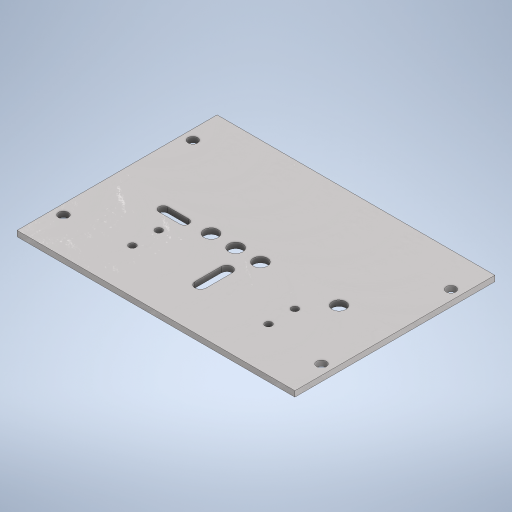
# Autodesk Inventor part: dach
Saved by Autodesk Inventor 2023 (Build 270158000, 158)
## iProperties
Created: 2023-07-07
Part Number: dach
Material: Stal miękka, spawana
Document SubType Name: Modeling
Designer: Kamil
Density: 7.85 g/cm^3
Appearance: Spawane — stal miękka
Author: Kamil
Autodesk Inventor part; units mm, degrees
ref_plane "YZ Plane" through (0, 0, 0) normal (1, 0, 0) x (0, 1, 0)
ref_plane "XZ Plane" through (0, 0, 0) normal (0, 1, 0) x (-1, 0, 0)
ref_plane "XY Plane" through (0, 0, 0) normal (0, 0, 1) x (1, 0, 0)
sketch "Szkic1" plane through (0, 0, 0) normal (0, 1, 0) x (-1, 0, 0)
  line L0 (0, 0) -> (-100, 0)
  line L1 (-100, 0) -> (-100, -70)
  line L2 (-100, -70) -> (0, -70)
  line L3 (0, -70) -> (0, 0)
  dimension "d0" = 100
  dimension "d1" = 70
  constraints: 8 end point, 2 parallel, 1 horizontal, 1 perpendicular
  measures "d0" distance of L2.end L1.end
  measures "d1" distance of L1.end L0.end
extrude "Wyciągnięcie proste1" add sketch "Szkic1" along normal blind 0.5
sketch "Szkic2" plane through (0, 0.5, 0) normal (0, 1, 0) x (1, 0, 0)
  line L0 (84.2801, 35.4995) -> (78.4801, 35.4995) projected
  line L1 (84.3801, 29.5995) -> (84.3801, 35.3995) projected
  line L2 (78.4801, 29.4995) -> (84.2801, 29.4995) projected
  line L3 (78.3801, 35.3995) -> (78.3801, 29.5995) projected
  circle A0 centre (53.6914, 31.8917) radius 2.05 projected
  circle A1 centre (44.8014, 31.8917) radius 2.05 projected
  circle A2 centre (35.9114, 31.8917) radius 2.05 projected
  line L4 (27.6783, 30.5334) -> (27.6783, 31.1734) projected
  line L5 (19.4183, 31.1734) -> (19.4183, 30.5334) projected
  line L6 (84.3801, 29.4995) -> (78.3801, 29.4995)
  line L7 (78.3801, 29.4995) -> (78.3801, 35.4995)
  line L8 (78.3801, 35.4995) -> (84.3801, 35.4995)
  line L9 (84.3801, 35.4995) -> (84.3801, 29.4995)
  line L10 (84.8801, 28.9995) -> (77.8801, 28.9995)
  line L11 (77.8801, 28.9995) -> (77.8801, 35.9995)
  line L12 (77.8801, 35.9995) -> (84.8801, 35.9995)
  line L13 (84.8801, 35.9995) -> (84.8801, 28.9995)
  circle A3 centre (53.6914, 31.8917) radius 2.55
  circle A4 centre (44.8014, 31.8917) radius 2.55
  circle A5 centre (35.9114, 31.8917) radius 2.55
  line L14 (27.6783, 30.5334) -> (19.4183, 30.5334)
  line L15 (19.4183, 30.5334) -> (19.4183, 31.1734)
  line L16 (19.4183, 31.1734) -> (27.6783, 31.1734)
  line L17 (27.6783, 31.1734) -> (27.6783, 30.5334)
  line L18 (28.9783, 32.4734) -> (18.1183, 32.4734)
  line L19 (18.1183, 32.4734) -> (18.1183, 29.2334)
  line L20 (18.1183, 29.2334) -> (28.9783, 29.2334)
  line L21 (28.9783, 29.2334) -> (28.9783, 32.4734)
  point P0 (0, 0)
  dimension "d4" = 0.5
  dimension "d5" = 0.5
  dimension "d6" = 0.5
  dimension "d7" = 0.5
  dimension "d8" = 1.3
  constraints: 32 end point, 8 parallel, 4 perpendicular, 3 centre point, 2 horizontal, 6 other
  measures "d4" distance between parallel lines of L9 L13
  measures "d5" radial gap between concentric circles of A0 A3
  measures "d6" radial gap between concentric circles of A1 A4
  measures "d7" radial gap between concentric circles of A2 A5
  measures "d8" distance between parallel lines of L16 L18
extrude "Wyciągnięcie proste2" cut sketch "Szkic2" against normal through all contours L8 L9 L1 L6 L2 L7 L3 L0 | A0 | A1 | A2 | L14 L5 L16 L4 | L10 L11 L12 L13 | A3 | A4 | A5 | L21 L20 L19 L18
sketch "Szkic3" plane through (0, 0.5, 0) normal (0, 1, 0) x (1, 0, 0)
  circle A0 centre (3.55, 57.7319) radius 1.5 projected
  circle A1 centre (3.55, 11.1233) radius 1.5 projected
  circle A2 centre (96.45, 57.7319) radius 1.5 projected
  circle A3 centre (96.45, 11.1233) radius 1.5 projected
  circle A4 centre (25.5, 23.5) radius 1 projected
  circle A5 centre (25.5, 14) radius 1 projected
  circle A6 centre (50, 23.5) radius 1 projected
  circle A7 centre (50, 14) radius 1 projected
  circle A8 centre (74.5, 23.5) radius 1 projected
  circle A9 centre (74.5, 14) radius 1 projected
  point P0 (0, 0)
extrude "Wyciągnięcie proste3" cut sketch "Szkic3" against normal through all
sketch "Szkic4" plane through (0, 0.5, 0) normal (0, 1, 0) x (1, 0, 0)
  circle A0 centre (3.55, 57.7319) radius 1.5 projected
  circle A1 centre (50, 14) radius 1 projected
  circle A2 centre (74.5, 14) radius 1 projected
  circle A3 centre (25.5, 23.5) radius 1 projected
  circle A4 centre (96.45, 57.7319) radius 1.5 projected
  circle A5 centre (3.55, 11.1233) radius 1.5 projected
  circle A6 centre (50, 23.5) radius 1 projected
  circle A7 centre (74.5, 23.5) radius 1 projected
  circle A8 centre (25.5, 14) radius 1 projected
  circle A9 centre (96.45, 11.1233) radius 1.5 projected
  circle A10 centre (44.8014, 31.8917) radius 2.55 projected
  circle A11 centre (35.9114, 31.8917) radius 2.55 projected
  circle A12 centre (53.6914, 31.8917) radius 2.55 projected
  line L0 (28.9783, 29.2334) -> (18.1183, 29.2334) projected
  line L1 (18.1183, 29.2334) -> (18.1183, 32.4734) projected
  line L2 (18.1183, 32.4734) -> (28.9783, 32.4734) projected
  line L3 (28.9783, 32.4734) -> (28.9783, 29.2334) projected
  line L4 (77.8801, 28.9995) -> (77.8801, 35.9995) projected
  line L5 (77.8801, 35.9995) -> (84.8801, 35.9995) projected
  line L6 (84.8801, 35.9995) -> (84.8801, 28.9995) projected
  line L7 (84.8801, 28.9995) -> (77.8801, 28.9995) projected
  line L8 (100, 0) -> (100, 70) projected
  line L9 (100, 70) -> (0, 70) projected
  line L10 (0, 70) -> (0, 0) projected
  line L11 (0, 0) -> (100, 0) projected
extrude "Wyciągnięcie proste4" add sketch "Szkic4" along normal blind 1.2
sketch "Szkic5" plane through (0, 1.7, 0) normal (0, 1, 0) x (1, 0, 0)
  circle A0 centre (25.5, 14) radius 1 projected
  line L0 (100, 70) -> (0, 70) projected
  line L1 (0, 70) -> (0, 0) projected
  line L2 (0, 0) -> (100, 0) projected
  line L3 (100, 0) -> (100, 70) projected
  circle A1 centre (53.6914, 31.8917) radius 2.55 projected
  circle A2 centre (44.8014, 31.8917) radius 2.55 projected
  circle A3 centre (25.5, 14) radius 1 projected
  circle A4 centre (3.55, 57.7319) radius 1.5 projected
  circle A5 centre (50, 14) radius 1 projected
  circle A6 centre (74.5, 14) radius 1 projected
  circle A7 centre (25.5, 23.5) radius 1 projected
  circle A8 centre (96.45, 57.7319) radius 1.5 projected
  circle A9 centre (3.55, 11.1233) radius 1.5 projected
  circle A10 centre (50, 23.5) radius 1 projected
  circle A11 centre (74.5, 23.5) radius 1 projected
  circle A12 centre (96.45, 11.1233) radius 1.5 projected
  circle A13 centre (35.9114, 31.8917) radius 2.55 projected
  line L4 (77.8801, 28.9995) -> (77.8801, 35.9995) projected
  line L5 (77.8801, 35.9995) -> (84.8801, 35.9995) projected
  line L6 (84.8801, 35.9995) -> (84.8801, 28.9995) projected
  line L7 (84.8801, 28.9995) -> (77.8801, 28.9995) projected
  line L8 (28.9783, 29.2334) -> (18.1183, 29.2334) projected
  line L9 (18.1183, 29.2334) -> (18.1183, 32.4734) projected
  line L10 (18.1183, 32.4734) -> (28.9783, 32.4734) projected
  line L11 (28.9783, 32.4734) -> (28.9783, 29.2334) projected
  circle A14 centre (3.55, 11.1233) radius 1.5 projected
  circle A15 centre (3.55, 11.1233) radius 1.75
  circle A16 centre (3.55, 57.7319) radius 1.5 projected
  circle A17 centre (3.55, 57.7319) radius 1.75
  circle A18 centre (96.45, 11.1233) radius 1.75
  circle A19 centre (96.45, 57.7319) radius 1.5 projected
  circle A20 centre (96.45, 57.7319) radius 1.75
  circle A21 centre (25.5, 14) radius 1 projected
  circle A22 centre (25.5, 14) radius 1.25
  circle A23 centre (25.5, 23.5) radius 1 projected
  circle A24 centre (25.5, 23.5) radius 1.25
  circle A25 centre (50, 23.5) radius 1 projected
  circle A26 centre (50, 23.5) radius 1.25
  circle A27 centre (50, 14) radius 1 projected
  circle A28 centre (50, 14) radius 1.25
  circle A29 centre (74.5, 23.5) radius 1 projected
  circle A30 centre (74.5, 23.5) radius 1.25
  circle A31 centre (74.5, 14) radius 1 projected
  circle A32 centre (74.5, 14) radius 1.25
  dimension "d15" = 3.5
  dimension "d16" = 3.5
  dimension "d17" = 3.5
  dimension "d18" = 3.5
  dimension "d19" = 2.5
  dimension "d20" = 2.5
  dimension "d21" = 2.5
  dimension "d22" = 2.5
  dimension "d23" = 2.5
  dimension "d24" = 2.5
  constraints: 10 centre point, 10 coincident
  measures "d15" diameter of A15
  measures "d16" diameter of A17
  measures "d17" diameter of A18
  measures "d18" diameter of A20
  measures "d19" diameter of A22
  measures "d20" diameter of A24
  measures "d21" diameter of A26
  measures "d22" diameter of A28
  measures "d23" diameter of A30
  measures "d24" diameter of A32
extrude "Wyciągnięcie proste5" cut sketch "Szkic5" against normal through all contours A0 | A4 | A5 | A6 | A7 | A8 | A9 | A10 | A11 | A12 | A15 | A17 | A18 | A20 | A22 | A24 | A26 | A28 | A30 | A32
sketch "Szkic6" plane through (0, 1.7, 0) normal (0, 1, 0) x (1, 0, 0)
  circle A0 centre (50, 23.5) radius 1.25 projected
  circle A1 centre (50, 14) radius 1.25 projected
  circle A2 centre (50, 14) radius 1.25 projected
  line L0 (50, 23.5) -> (50, 14) construction
  line L1 (52, 23.5) -> (52, 14)
  line L2 (48, 14) -> (48, 23.5)
  arc A3 (52, 23.5) -> (48, 23.5) centre (50, 23.5) ccw
  arc A4 (48, 14) -> (52, 14) centre (50, 14) ccw
  point P0 (0, 0)
  point P1 (50, 18.75)
  constraints: 8 end point, 4 point on circle, 4 tangent, 2 centre point, 1 midpoint, 1 parallel
extrude "Wyciągnięcie proste6" cut sketch "Szkic6" against normal through all contours A0 | A1 | L1 A4 L2 A3
sketch "Szkic7" plane through (0, 1.7, 0) normal (0, 1, 0) x (1, 0, 0)
  arc A0 (52, 23.5) -> (48, 23.5) centre (50, 23.5) ccw projected
  line L0 (52, 23.5) -> (52, 14) projected
  arc A1 (48, 14) -> (52, 14) centre (50, 14) ccw projected
  line L1 (48, 14) -> (48, 23.5) projected
  circle A2 centre (25.5, 23.5) radius 1.25 projected
  circle A3 centre (74.5, 23.5) radius 1.25 projected
  circle A4 centre (96.45, 57.7319) radius 1.75 projected
  circle A5 centre (3.55, 11.1233) radius 1.75 projected
  circle A6 centre (25.5, 14) radius 1.25 projected
  circle A7 centre (74.5, 14) radius 1.25 projected
  circle A8 centre (96.45, 11.1233) radius 1.75 projected
  circle A9 centre (3.55, 57.7319) radius 1.75 projected
  line L2 (100, 70) -> (0, 70) projected
  line L3 (0, 70) -> (0, 0) projected
  line L4 (0, 0) -> (100, 0) projected
  line L5 (100, 0) -> (100, 70) projected
  circle A10 centre (53.6914, 31.8917) radius 2.55 projected
  circle A11 centre (44.8014, 31.8917) radius 2.55 projected
  circle A12 centre (35.9114, 31.8917) radius 2.55 projected
  line L6 (77.8801, 28.9995) -> (77.8801, 35.9995) projected
  line L7 (77.8801, 35.9995) -> (84.8801, 35.9995) projected
  line L8 (84.8801, 35.9995) -> (84.8801, 28.9995) projected
  line L9 (84.8801, 28.9995) -> (77.8801, 28.9995) projected
  line L10 (28.9783, 29.2334) -> (18.1183, 29.2334) projected
  line L11 (18.1183, 29.2334) -> (18.1183, 32.4734) projected
  line L12 (18.1183, 32.4734) -> (28.9783, 32.4734) projected
  line L13 (28.9783, 32.4734) -> (28.9783, 29.2334) projected
extrude "Wyciągnięcie proste7" add sketch "Szkic7" along normal blind 0.3
sketch "Szkic8" plane through (0, 2, 0) normal (0, 1, 0) x (1, 0, 0)
  line L0 (0, 0) -> (100, 0) projected
  line L1 (100, 0) -> (0, 0)
  line L2 (0, 0) -> (0, -2)
  line L3 (0, -2) -> (100, -2)
  line L4 (100, -2) -> (100, 0)
  dimension "d31" = 2
  constraints: 8 end point, 2 parallel, 1 horizontal, 1 perpendicular
  measures "d31" distance of L2.end L1.end
extrude "Wyciągnięcie proste8" add sketch "Szkic8" against normal blind 2
sketch "Szkic9" plane through (0, 2, 0) normal (0, 1, 0) x (1, 0, 0)
  line L0 (28.9783, 32.4734) -> (28.9783, 29.2334) projected
  line L1 (18.1183, 29.2334) -> (18.1183, 32.4734) projected
  line L2 (18.1183, 32.4734) -> (28.9783, 32.4734) projected
  line L3 (28.9783, 29.2334) -> (18.1183, 29.2334) projected
  line L4 (18.1183, 30.8534) -> (28.9783, 30.8534) construction
  line L5 (19.7383, 32.4734) -> (27.3583, 32.4734)
  line L6 (27.3583, 29.2334) -> (19.7383, 29.2334)
  arc A0 (19.7383, 32.4734) -> (19.7383, 29.2334) centre (19.7383, 30.8534) ccw
  arc A1 (27.3583, 29.2334) -> (27.3583, 32.4734) centre (27.3583, 30.8534) ccw
  point P0 (0, 0)
  point P1 (23.5483, 30.8534)
  constraints: 8 end point, 6 point on circle, 4 tangent, 3 midpoint, 2 centre point, 2 point on line, 1 parallel
extrude "Wyciągnięcie proste9" add sketch "Szkic9" against normal up to surface (2 mm away) contours L0 A1 L2 | L0 L3 A1 | A0 L1 L2 | L3 L1 A0
sketch "Szkic10" plane through (0, 2, 0) normal (0, 1, 0) x (1, 0, 0)
  line L0 (77.8801, 35.9995) -> (84.8801, 35.9995) projected
  line L1 (84.8801, 35.9995) -> (84.8801, 28.9995) projected
  line L2 (84.8801, 28.9995) -> (77.8801, 28.9995) projected
  line L3 (77.8801, 28.9995) -> (77.8801, 35.9995) projected
  circle A0 centre (81.3801, 32.4995) radius 2.5
  point P0 (0, 0)
  dimension "d36" = 5
  constraints: 1 centre point
  measures "d36" diameter of A0
extrude "Wyciągnięcie proste10" add sketch "Szkic10" against normal up to surface (2 mm away)
